magnet-mounter v11 (Autodesk Fusion 360 design; units mm, degrees)
Autodesk Fusion 360 part; units mm, degrees
sketch "スケッチ1" plane through (0, 0, 0) normal (0, 0, 1) x (1, 0, 0)
  circle A0 centre (0, 0) radius 0.75
  circle A1 centre (0, 0) radius 1
  circle A2 centre (0, 0) radius 1.5
  circle A3 centre (0, 0) radius 1.25
  dimension "d1" = 1.5
  dimension "d2" = 2
  dimension "d3" = 3
  dimension "d9" = 2.5
  measures "d1" diameter of A0
  measures "d2" diameter of A1
  measures "d3" diameter of A2
  measures "d9" diameter of A3
extrude "押し出し1" add sketch "スケッチ1" against normal blind 1 contours A1 | A3
extrude "押し出し2" add sketch "スケッチ1" along normal blind 2 contours A2 | A3
extrude "押し出し3" add sketch "スケッチ1" against normal blind 0.5 contours A1 | A2 | A3
